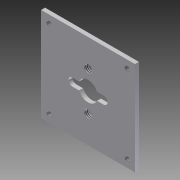
# Autodesk Inventor part: Slide Plate BD Motor mount
Saved by Autodesk Inventor 2012 (Build 160160000, 160)
## iProperties
Created: 2012-06-30
Part Number: Slide Plate BD Motor mount
Material: Default
Document SubType Name: Modeling
Designer: Bruce
Density: 1 g/cm^3
Author: Bruce
Autodesk Inventor part; units mm, degrees
ref_plane "YZ Plane" through (0, 0, 0) normal (1, 0, 0) x (0, 1, 0)
ref_plane "XZ Plane" through (0, 0, 0) normal (0, 1, 0) x (-1, 0, 0)
ref_plane "XY Plane" through (0, 0, 0) normal (0, 0, 1) x (1, 0, 0)
sketch "Sketch1" plane through (0, 0, 0) normal (0, 0, 1) x (1, 0, 0)
  line L0 (-38.1, 38.1) -> (38.1, 38.1)
  line L1 (38.1, 38.1) -> (38.1, -38.1)
  line L2 (38.1, -38.1) -> (-38.1, -38.1)
  line L3 (-38.1, -38.1) -> (-38.1, 38.1)
  circle A0 centre (0, 0) radius 7.9375
  line L4 (38.1, 38.1) -> (50.8, 38.1)
  line L5 (50.8, 38.1) -> (50.8, -38.1)
  line L6 (50.8, -38.1) -> (38.1, -38.1)
  line L7 (38.1, -38.1) -> (38.1, 38.1)
  line L8 (-38.1, 38.1) -> (-50.8, 38.1)
  line L9 (-50.8, 38.1) -> (-50.8, -38.1)
  line L10 (-50.8, -38.1) -> (-38.1, -38.1)
  line L11 (-38.1, -38.1) -> (-38.1, 38.1)
  arc A1 (-13.97, 3.175) -> (-13.97, -3.175) centre (-13.97, 0) ccw
  arc A2 (13.97, -3.175) -> (17.145, 0) centre (13.97, 0) ccw
  line L12 (-13.97, 3.175) -> (13.97, 3.175)
  arc A3 (17.145, 0) -> (13.97, 3.175) centre (13.97, 0) ccw
  line L13 (-13.97, -3.175) -> (13.97, -3.175)
  circle A4 centre (0, 15.875) radius 3.175
  circle A5 centre (0, -15.875) radius 3.175
  point P0 (-31.75, 31.75)
  point P1 (31.75, 31.75)
  point P2 (31.75, -31.75)
  point P3 (-31.75, -31.75)
  dimension "d0" = 76.2
  dimension "d1" = 76.2
  dimension "d2" = 38.1
  dimension "d3" = 38.1
  dimension "d4" = 15.875
  dimension "d5" = 6.35
  dimension "d6" = 6.35
  dimension "d7" = 6.35
  dimension "d8" = 6.35
  dimension "d36" = 12.7
  dimension "d37" = 12.7
  dimension "d42" = 6.35
  dimension "d43" = 27.94
  dimension "d44" = 3.175
  dimension "d45" = 13.97
  dimension "d46" = 6.35
  dimension "d47" = 6.35
  dimension "d48" = 15.875
  dimension "d49" = 31.75
  constraints: 28 end point, 7 parallel, 7 point on circle, 6 centre point, 4 horizontal, 4 tangent, 4 vertical alignment, 3 horizontal alignment, 3 perpendicular, 2 collinear, 1 coincident
  measures "d0" distance of L2.end L0.start
  measures "d1" distance of L1.end L2.end
  measures "d2" distance from line of L3 point (0, 0)
  measures "d3" distance from line of point (0, 0) L2
  measures "d4" diameter of A0
  measures "d5" distance from line of L0 point (-31.75, 31.75)
  measures "d6" distance from line of L3 point (-31.75, 31.75)
  measures "d7" distance from line of point (31.75, 31.75) L1
  measures "d8" distance from line of L2 point (-31.75, -31.75)
  measures "d36" distance of L0.end L4.end
  measures "d37" distance of L0.start L8.end
  measures "d42" diameter of A1
  measures "d43" distance of A2.centre A1.centre
  measures "d44" radius of A3
  measures "d45" distance of point (0, 0) A1.centre
  measures "d46" diameter of A5
  measures "d47" diameter of A4
  measures "d48" distance of A5.centre point (0, 0)
  measures "d49" distance of A5.centre A4.centre
extrude "Extrusion1" add sketch "Sketch1" against normal blind 3.175 contours L0 L1 L2 L3 | A0 L12 A3 A2 L13 | A0 L13 A1 L12 | A4 | A5
hole "Hole1" at (-31.75, 31.75, 0) at (31.75, 31.75, 0) at (31.75, -31.75, 0) at (-31.75, -31.75, 0) direction (0, 0, -1) diameter 3.9624 end through all thread size "10-32 UNF" class "2B" standard "ANSI Unified Screw Threads"
extrude "Extrusion3" cut sketch "Sketch1" against normal through all contours A0 L13 L12 | A0 L12 A3 A2 L13 | A0 L13 A1 L12 | A4 | A5
thread "Thread1" size "1/4-20 UNC" class "2B" standard "ANSI Unified Screw Threads" full length
thread "Thread2" size "1/4-20 UNC" class "2B" standard "ANSI Unified Screw Threads" full length
equation "\"d2\" = 0.5 * d1"
equation "\"d3\" = 0.5 * d0"
equation "\"d7\" = d6"
equation "\"d8\" = d5"
equation "\"d45\" = 0.5 * d43"
equation "\"d48\" = 0.5 * d49"
body "Solid1"
